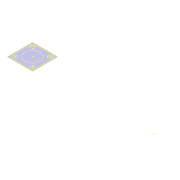
# Autodesk Inventor part: 30_CUBE_openSIM_Lensholder_THORLABSrods
Saved by Autodesk Inventor 2019 (Build 230136000, 136)
## iProperties
Created: 2019-10-13
Part Number: 30_CUBE_openSIM_Lensholder_THORLABSrods
Material: Generic
Document SubType Name: Modeling
Designer: diederichbenedict
Density: 1 g/cm^3
Appearance: Default
Author: diederichbenedict
Autodesk Inventor part; units mm, degrees
ref_plane "YZ Plane" through (0, 0, 0) normal (1, 0, 0) x (0, 1, 0)
ref_plane "XZ Plane" through (0, 0, 0) normal (0, 1, 0) x (-1, 0, 0)
ref_plane "XY Plane" through (0, 0, 0) normal (0, 0, 1) x (1, 0, 0)
ref_plane "Work Plane1" through (-266.5502, -274.7073, -10.9919) normal (0, -1, 0) x (0, 0, -1)
sketch "Sketch1" plane through (-266.5502, -274.7073, -10.9919) normal (0, -1, 0) x (0, 0, -1)
  line L0 (-20.066, 62.7742) -> (-20.066, 26.9166) construction
  line L1 (-20.066, 26.9166) -> (-17.9288, 24.7794) construction
  line L2 (-17.9288, 24.7794) -> (17.9288, 24.7794) construction
  line L3 (17.9288, 24.7794) -> (20.066, 26.9166) construction
  line L4 (20.066, 26.9166) -> (20.066, 62.7742) construction
  line L5 (20.066, 62.7742) -> (17.9288, 64.9114) construction
  line L6 (17.9288, 64.9114) -> (-17.9288, 64.9114) construction
  line L7 (-17.9288, 64.9114) -> (-20.066, 62.7742) construction
  circle A0 centre (15, 29.8455) radius 3.2639 construction
  circle A1 centre (15, 59.8454) radius 3.2639 construction
  circle A2 centre (-15, 59.8454) radius 3.2639 construction
  circle A3 centre (-15, 29.8455) radius 3.2639 construction
  circle A4 centre (0, 44.8454) radius 13.3985 construction
  circle A5 centre (15, 59.8454) radius 3 construction
  circle A6 centre (15, 29.8455) radius 3 construction
  circle A7 centre (0, 44.8454) radius 15
  line L8 (-20.066, 24.7794) -> (9.631, 24.7794)
  line L9 (9.631, 24.7794) -> (9.631, 64.9114)
  line L10 (9.631, 64.9114) -> (-20.066, 64.9114)
  line L11 (-20.066, 64.9114) -> (-20.066, 24.7794)
  circle A8 centre (-15, 29.8455) radius 3.15
  circle A9 centre (-15, 59.8454) radius 3.15
  point P0 (-10.9919, 266.5502)
  point P1 (9.631, 33.3457)
  point P2 (9.631, 56.3451)
  dimension "d0" = 30
  dimension "d6" = 6.3
  dimension "d7" = 6.3
  constraints: 8 end point, 3 centre point, 3 point on line, 2 parallel, 2 point on circle, 1 coincident, 1 horizontal, 1 perpendicular
  measures "d0" diameter of A7
  measures "d6" diameter of A8
  measures "d7" diameter of A9
extrude "Extrusion1" add sketch "Sketch1" along normal blind 10 contours A7 L9 L8 L11 L10
fillet "Fillet1" radius 3 6 edges at (-241.7708, -279.7073, 9.0741) (-201.6388, -279.7073, 9.0741) (-241.7708, -279.7073, -20.623) (-201.6388, -279.7073, -20.623) (-210.2051, -279.7073, -20.623) (-233.2045, -279.7073, -20.623)
body "Solid1"
